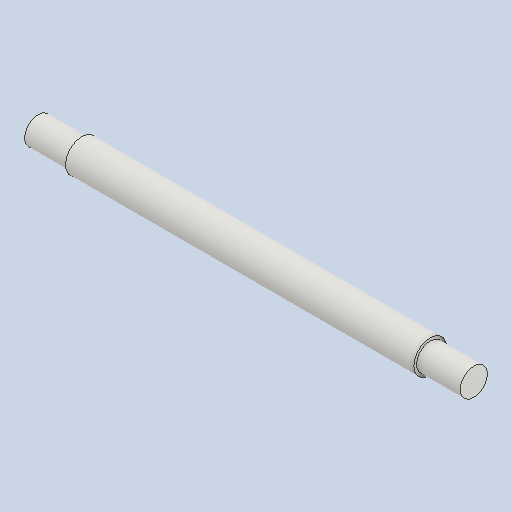
# Autodesk Inventor part: Shaft
Saved by Autodesk Inventor 2024 (Build 280153000, 153)
## iProperties
CustomPartVersion: 1
Created: 2023-11-21
Part Number: Shaft
Material: Steel
Document SubType Name: Modeling
Designer: Greg
Density: 1 g/cm^3
Appearance: Steel
Length: 2.500 in
Author: Greg
Autodesk Inventor part; units mm, degrees
ref_plane "Start Plane" through (0, 0, 0) normal (1, 0, 0) x (0, 1, 0)
ref_plane "XZ Plane" through (0, 0, 0) normal (0, 1, 0) x (-1, 0, 0)
ref_plane "XY Plane" through (0, 0, 0) normal (0, 0, 1) x (1, 0, 0)
sketch "Main Sketch" plane through (0, 0, 0) normal (0, 0, 1) x (1, 0, 0)
  line L0 (0, 0) -> (63.5, 0)
  line L1 (0, 0) -> (0, 1.9844)
  line L2 (0, 1.9844) -> (6.35, 1.9844)
  line L3 (6.35, 1.9844) -> (6.35, 2.3813)
  line L4 (57.15, 2.3813) -> (57.15, 1.9844)
  line L5 (6.35, 2.3813) -> (57.15, 2.3813)
  line L6 (63.5, 1.9844) -> (63.5, 0)
  line L7 (57.15, 1.9844) -> (63.5, 1.9844)
  dimension "d3" = 3.9688
  dimension "d4" = 4.7625
  dimension "d5" = 3.9688
  constraints: 16 end point, 4 vertical, 3 horizontal
  measures "d3" diameter of L2 L0
  measures "d4" diameter of L5 L0
  measures "d5" diameter of L7 L0
revolve "Revolution1" add sketch "Main Sketch" angle 360 about axis through (0, 0, 0) along (1, 0, 0)
equation "\"Length\" = 63.5"
body "Solid1"
